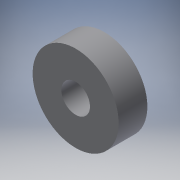
# Autodesk Inventor part: Bearing
Saved by Autodesk Inventor 2019 (Build 230136000, 136)
## iProperties
Created: 2020-01-19
Part Number: Bearing
Material: Generic
Document SubType Name: Modeling
Designer: peter
Density: 7.46039 g/cm^3
Appearance: Default
Mass: 3 g
Surface Area: 4.02124 cm^2
Volume: 0.402124 cm^3
Author: peter
Autodesk Inventor part; units mm, degrees
ref_plane "YZ Plane" through (0, 0, 0) normal (1, 0, 0) x (0, 1, 0)
ref_plane "XZ Plane" through (0, 0, 0) normal (0, 1, 0) x (-1, 0, 0)
ref_plane "XY Plane" through (0, 0, 0) normal (0, 0, 1) x (1, 0, 0)
sketch "Sketch1" plane through (0, 0, 0) normal (0, 0, 1) x (1, 0, 0)
  circle A0 centre (1.2337, 1.1676) radius 2
  circle A1 centre (1.2337, 1.1676) radius 6
  point P0 (0, 0)
  dimension "d0" = 4
  dimension "d1" = 12
  constraints: 2 centre point, 1 coincident
  measures "d0" diameter of A0
  measures "d1" diameter of A1
extrude "Extrusion1" add sketch "Sketch1" along normal blind 4
body "Solid1"
